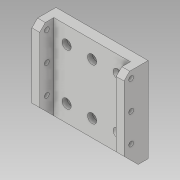
# Autodesk Inventor part: complex_cube_plane
Saved by Autodesk Inventor 2017 (Build 210142000, 142)
## iProperties
Part Number: complex_cube_plane
Material: Aluminium 6061
Document SubType Name: Modeling
Designer: Max
Density: 2.7 g/cm^3
Appearance: Vorgabe
Mass: 86.6412 g
Surface Area: 126.297 cm^2
Volume: 32.0893 cm^3
Author: Max
Autodesk Inventor part; units mm, degrees
ref_plane "YZ Plane" through (0, 0, 0) normal (1, 0, 0) x (0, 1, 0)
ref_plane "XZ Plane" through (0, 0, 0) normal (0, 1, 0) x (-1, 0, 0)
ref_plane "XY Plane" through (0, 0, 0) normal (0, 0, 1) x (1, 0, 0)
sketch "Skizze1" plane through (0, 0, 0) normal (0, 1, 0) x (-1, 0, 0)
  line L0 (-32.5, 30) -> (32.5, 30)
  line L1 (32.5, 30) -> (32.5, -30)
  line L2 (32.5, -30) -> (-32.5, -30)
  line L3 (-32.5, -30) -> (-32.5, 30)
  line L4 (-32.5, 30) -> (32.5, -30) construction
  line L5 (32.5, 30) -> (-32.5, -30) construction
  point P0 (0, 0)
  dimension "d0" = 65
  dimension "d1" = 60
  constraints: 12 end point, 2 midpoint, 2 parallel, 1 horizontal, 1 perpendicular
  measures "d0" distance of L1.end L2.end
  measures "d1" distance of L0.end L1.end
extrude "Extrusion1" add sketch "Skizze1" along normal blind 7
sketch "Skizze2" plane through (0, 7, 0) normal (0, 1, 0) x (1, 0, 0)
  line L0 (24.5, -20) -> (-24.5, -20)
  line L1 (-24.5, -20) -> (-24.5, 20)
  line L2 (-24.5, 20) -> (24.5, 20)
  line L3 (24.5, 20) -> (24.5, -20)
  line L4 (24.5, -20) -> (-24.5, 20) construction
  line L5 (-24.5, -20) -> (24.5, 20) construction
  line L6 (29.8936, 0) -> (-30.3656, 0) construction
  point P0 (0, 0)
  point P1 (0, 0)
  point P2 (-24.5, 0)
  point P3 (24.5, 0)
  dimension "d4" = 49
  dimension "d5" = 40
  constraints: 14 end point, 5 midpoint, 3 point on line, 2 horizontal, 2 parallel, 1 perpendicular
  measures "d4" distance of L1.end L2.end
  measures "d5" distance of L0.end L1.end
hole "Bohrung1" [suppressed]
sketch "Skizze3" plane through (0, 0, 0) normal (0, -1, 0) x (1, 0, 0)
  line L0 (-18, -18) -> (18, -18)
  line L1 (18, -18) -> (18, 18)
  line L2 (18, 18) -> (-18, 18)
  line L3 (-18, 18) -> (-18, -18)
  line L4 (-18, -18) -> (18, 18) construction
  line L5 (18, -18) -> (-18, 18) construction
  line L6 (0, -22.3415) -> (0, 25.3309) construction
  point P0 (0, 0)
  point P1 (0, 18)
  point P2 (0, -18)
  dimension "d13" = 36
  dimension "d14" = 36
  constraints: 14 end point, 4 midpoint, 2 parallel, 2 point on line, 1 horizontal, 1 perpendicular, 1 vertical
  measures "d13" distance of L2.end L1.end
  measures "d14" distance of L0.end L1.end
hole "Bohrung2" at (0, 0, 18) at (0, 0, -18) at (-18, 0, 18) at (-18, 0, -18) at (18, 0, 18) at (18, 0, -18) direction (0, 1, 0) diameter 3.4 depth 8 tip angle 118 counterbore diameter 6.5 counterbore depth 3.4 clearance for "Inbusschraube ISO 4762" size "M3" standard "ISO"
sketch "Skizze4" plane through (0, 0, 0) normal (0, -1, 0) x (1, 0, 0)
  circle A0 centre (18, 18) radius 3.25 projected
  circle A1 centre (-18, 18) radius 3.25 projected
  circle A2 centre (0, 18) radius 3.25 projected
  circle A3 centre (0, -18) radius 3.25 projected
  circle A4 centre (-18, -18) radius 3.25 projected
  circle A5 centre (18, -18) radius 3.25 projected
  line L0 (32.5, 30) -> (-32.5, 30) projected
  line L1 (-32.5, 30) -> (-32.5, -30) projected
  line L2 (-32.5, -30) -> (32.5, -30) projected
  line L3 (32.5, -30) -> (32.5, 30) projected
  line L4 (-32.5, 30) -> (-27, 30)
  line L5 (-27, 30) -> (-27, -30)
  line L6 (-27, -30) -> (-32.5, -30)
  line L7 (-32.5, -30) -> (-32.5, 30)
  line L8 (32.5, -30) -> (-32.5, -30) projected
  line L9 (27, -30) -> (32.5, -30)
  line L10 (32.5, -30) -> (32.5, 30)
  line L11 (32.5, 30) -> (27, 30)
  line L12 (27, 30) -> (27, -30)
  point P0 (0, 0)
  dimension "d22" = 54
  dimension "d23" = 65
  dimension "d24" = 5.5
  constraints: 16 end point, 4 parallel, 2 horizontal, 2 perpendicular, 2 point on line
  measures "d22" distance between parallel lines of L12 L5
  measures "d23" distance between parallel lines of L3 L1
  measures "d24" distance of L0.end L4.end
extrude "Extrusion2" add sketch "Skizze4" along normal blind 10 contours L3 L2 L12 L0 | L5 L2 L1 L0
sketch "Skizze5" plane through (-32.5, 7, -30) normal (-1, 0, 0) x (0, 0, 1)
  line L0 (0, -7) -> (60, -7) projected
  line L1 (0, -7) -> (0, -17) projected
  line L2 (60, -17) -> (0, -17) projected
  line L3 (60, -7) -> (60, -17) projected
  point P0 (30, -7)
  point P1 (35, -12)
  dimension "d27" = 5
  dimension "d41" = 35
  dimension "d42" = 60
  measures "d27" distance from line of point (35, -12) L0
  measures "d41" distance from line of L1 point (35, -12)
  measures "d42" distance of L2.start L1.end
hole "Bohrung3" at (-32.5, -5, 5) direction (1, 0, 0) diameter 3.4 end through all clearance for "Inbusschraube ISO 4762" size "M3" standard "ISO"
pattern_linear "Rechteckige Anordnung1" count 3 spacing 20 along (0, 0, -1) of "Bohrung3" first direction both ways yes
chamfer "Fase2" distance 10 angle 45 2 edges at (-29.75, -10, -30) (29.75, -10, -30)
chamfer "Fase3" distance 4 angle 45 2 edges at (-29.75, -10, 30) (29.75, -10, 30)
equation "\"d24\" = -0.5 * d22 + 0.5 * d23"
